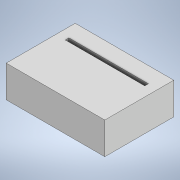
# Autodesk Inventor part: sunroof_motor_cover_clip_retention_patch
Saved by Autodesk Inventor 2021 (Build 250183000, 183)
## iProperties
Created: 2022-01-18
Part Number: sunroof_motor_cover_clip_retention_patch
Material: Generic
Document SubType Name: Modeling
Designer: Andrew
Density: 1 g/cm^3
Appearance: Default
Author: Andrew
Autodesk Inventor part; units mm, degrees
ref_plane "YZ Plane" through (0, 0, 0) normal (1, 0, 0) x (0, 1, 0)
ref_plane "XZ Plane" through (0, 0, 0) normal (0, 1, 0) x (-1, 0, 0)
ref_plane "XY Plane" through (0, 0, 0) normal (0, 0, 1) x (1, 0, 0)
sketch "Sketch1" plane through (0, 0, 0) normal (0, 1, 0) x (-1, 0, 0)
  line L0 (10.075, 7.05) -> (-10.075, 7.05)
  line L1 (-10.075, 7.05) -> (-10.075, -7.05)
  line L2 (-10.075, -7.05) -> (10.075, -7.05)
  line L3 (10.075, -7.05) -> (10.075, 7.05)
  line L4 (10.075, 7.05) -> (-10.075, -7.05) construction
  line L5 (-10.075, 7.05) -> (10.075, -7.05) construction
  line L6 (9.075, 6.05) -> (-9.075, 6.05)
  line L7 (-9.075, 6.05) -> (-9.075, -6.05)
  line L8 (-9.075, -6.05) -> (9.075, -6.05)
  line L9 (9.075, -6.05) -> (9.075, 6.05)
  line L10 (9.075, 6.05) -> (-9.075, -6.05) construction
  line L11 (-9.075, 6.05) -> (9.075, -6.05) construction
  line L12 (8.125, -3.075) -> (-8.125, -3.075)
  line L13 (-8.125, -3.075) -> (-8.125, -3.825)
  line L14 (-8.125, -3.825) -> (8.125, -3.825)
  line L15 (8.125, -3.825) -> (8.125, -3.075)
  line L16 (8.125, -3.075) -> (-8.125, -3.825) construction
  line L17 (-8.125, -3.075) -> (8.125, -3.825) construction
  point P0 (0, 0)
  point P1 (0, -3.45)
  point P2 (0, -3.45)
  point P3 (0, 0)
  dimension "d0" = 18.15
  dimension "d1" = 1
  dimension "d2" = 1
  dimension "d3" = 12.1
  dimension "d4" = 16.25
  dimension "d5" = 0.75
  dimension "d6" = 9.5
  constraints: 36 end point, 8 midpoint, 6 parallel, 3 horizontal, 3 perpendicular, 1 vertical alignment
  measures "d0" distance of L7.end L8.end
  measures "d1" distance between parallel lines of L2 L8
  measures "d2" distance between parallel lines of L1 L7
  measures "d3" distance of L6.end L7.end
  measures "d4" distance of L13.end L14.end
  measures "d5" distance of L14.end L12.start
  measures "d6" distance from line of L6 point (0, -3.45)
sketch "Sketch2" plane through (0, 0, 0) normal (1, 0, 0) x (0, 1, 0)
  line L0 (-2.4, 6.05) -> (-4.5, 6.05)
  line L1 (-4.5, 6.05) -> (-2.4, 4.05)
  line L2 (-2.4, 4.05) -> (-2.4, 6.05)
  line L3 (-2.4, -6.05) -> (-2.4, -4.05)
  line L4 (-2.4, -4.05) -> (-4.5, -6.05)
  line L5 (-4.5, -6.05) -> (-2.4, -6.05)
  point P0 (0, 0)
  point P1 (0, 6.05)
  point P2 (0, 6.05)
  point P3 (0, 6.05)
  point P4 (0, -6.05)
  point P5 (0, -6.05)
  point P6 (0, -6.05)
  dimension "d11" = 2
  dimension "d12" = 2
  dimension "d13" = 4.5
  dimension "d14" = 4.5
  dimension "d15" = 2.4
  constraints: 12 end point, 2 perpendicular, 2 point on line, 1 collinear, 1 horizontal, 1 vertical
  measures "d11" distance of L1.end L0.start
  measures "d12" distance of L3.start L3.end
  measures "d13" horizontal distance of point (0, 0) L0.end
  measures "d14" horizontal distance of point (0, 0) L4.end
  measures "d15" distance from line of point (0, 0) L3
extrude "Extrusion1" add sketch "Sketch1" along normal blind 2 contours L3 L2 L1 L0 | L9 L8 L7 L6
extrude "Extrusion2" add sketch "Sketch1" against normal blind 4.5 contours L3 L2 L1 L0
equation "\"d13\" = d9"
equation "\"d14\" = d9"
equation "\"d9\" = 4.5"
body "Solid1"
